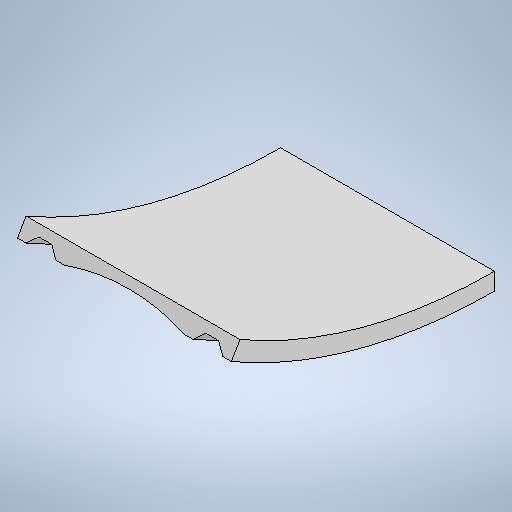
# Autodesk Inventor part: wheel_plate
Saved by Autodesk Inventor 2026.2 (Build 302298000, 298)
## iProperties
Created: 2026-01-18
Part Number: wheel_plate
Material: Generic
Document SubType Name: Modeling
Designer: gakut
Density: 1 g/cm^3
Appearance: Default
Author: gakut
Autodesk Inventor part; units mm, degrees
ref_plane "YZ Plane" through (0, 0, 0) normal (1, 0, 0) x (0, 1, 0)
ref_plane "XZ Plane" through (0, 0, 0) normal (0, 1, 0) x (-1, 0, 0)
ref_plane "XY Plane" through (0, 0, 0) normal (0, 0, 1) x (1, 0, 0)
sketch "Sketch2" plane through (0, 0, 0) normal (0, 0, 1) x (1, 0, 0)
  line L0 (-125, -5) -> (125, -5)
  line L1 (125, -5) -> (125, 5)
  line L2 (125, 5) -> (-125, 5)
  line L3 (-125, 5) -> (-125, -5)
  line L4 (-125, -5) -> (125, 5) construction
  line L5 (125, -5) -> (-125, 5) construction
  line L6 (-90, -5) -> (-80, -15)
  line L7 (80, -15) -> (90, -5)
  arc A0 (70, -15) -> (-70, -15) centre (0, -255) ccw
  line L8 (-80, -15) -> (-70, -15)
  line L9 (70, -15) -> (80, -15)
  line L10 (105, -5) -> (115, -15)
  line L11 (115, -15) -> (125, -15)
  line L12 (125, -15) -> (125, -5)
  line L13 (-105, -5) -> (-115, -15)
  line L14 (-115, -15) -> (-125, -15)
  line L15 (-125, -15) -> (-125, -5)
  point P0 (0, 0)
  dimension "d10" = 250
  dimension "d15" = 45
  dimension "d16" = 45
  dimension "d17" = 10
  dimension "d18" = 10
  dimension "d19" = 10
  dimension "d25" = 45
  dimension "d26" = 45
  dimension "d27" = 10
  dimension "d28" = 10
  dimension "d29" = 15
  dimension "d30" = 15
  dimension "d31" = 10
  constraints: 32 end point, 5 horizontal, 4 equal length, 4 point on line, 3 collinear, 2 midpoint, 2 point on circle, 1 centre point, 1 perpendicular, 1 tangent
  measures "d10" distance of L1.end L2.end
  measures "d15" angle of L0 L6
  measures "d16" angle of L0 L7
  measures "d17" distance of L8.end L6.end
  measures "d18" distance of L7.start L9.start
  measures "d19" distance between parallel lines of L0 L8
  measures "d25" angle of L10 L0
  measures "d26" angle of L13 L0
  measures "d27" distance of L10.end L11.end
  measures "d28" distance of L13.end L14.end
  measures "d29" distance of L6.start L13.start
  measures "d30" distance of L10.start L7.end
  measures "d31" distance between parallel lines of L0 L2
sketch "Sketch3" plane through (0, 0, 0) normal (1, 0, 0) x (0, 1, 0)
  arc A0 (80.384758, 300) -> (0, 0) centre (600, 0) ccw
  line L0 (600, 0) -> (0, 0) construction
  line L1 (80.384758, 300) -> (600, 0) construction
  dimension "d20" = 600
  dimension "d21" = 30
  dimension "d22" = 310.58285
  constraints: 4 end point, 2 point on circle, 1 centre point, 1 horizontal
  measures "d20" distance of L0.end L0.start
  measures "d21" angle of L0 L1
  measures "d22" distance of L0.end L1.start
sweep "Sweep1" add profiles "Sketch2" path "Sketch3"
equation "\"d15\" = d26"
equation "\"d16\" = d26"
equation "\"d17\" = d28"
equation "\"d18\" = d17"
equation "\"d25\" = d26"
equation "\"d27\" = d28"
equation "\"d30\" = d29"
body "Solid2"
